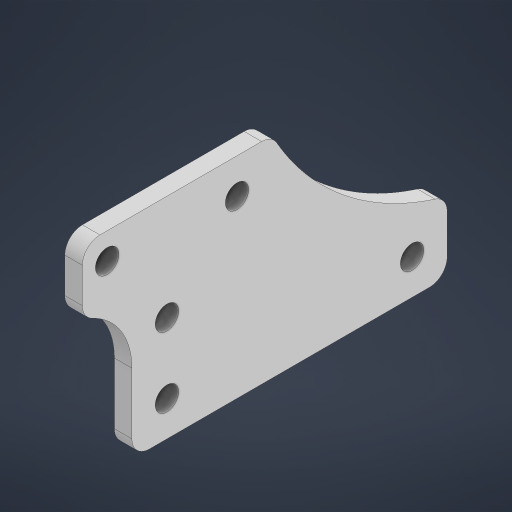
# Autodesk Inventor part: sled mounts
Saved by Autodesk Inventor 2024 (Build 280153000, 153)
## iProperties
Created: 2024-03-28
Part Number: sled mounts
Material: Generic
Document SubType Name: Modeling
Designer: Andrew
Density: 1 g/cm^3
Appearance: Default
Author: Andrew
Autodesk Inventor part; units mm, degrees
ref_plane "YZ Plane" through (0, 0, 0) normal (1, 0, 0) x (0, 1, 0)
ref_plane "XZ Plane" through (0, 0, 0) normal (0, 1, 0) x (-1, 0, 0)
ref_plane "XY Plane" through (0, 0, 0) normal (0, 0, 1) x (1, 0, 0)
sketch "Sketch1" plane through (0, 0, 0) normal (1, 0, 0) x (0, 1, 0)
  line L0 (0, 0) -> (12.7, 0)
  circle A0 centre (12.7, 0) radius 2.1209
  circle A1 centre (0, 0) radius 2.1209
  line L1 (12.7, 0) -> (12.7, 6.35)
  line L2 (12.7, 6.35) -> (19.05, 6.35)
  line L3 (19.05, 6.35) -> (-6.35, 6.35)
  line L4 (-6.35, 6.35) -> (-6.35, -6.35)
  line L5 (-6.35, -6.35) -> (19.05, -6.35)
  line L6 (19.05, -6.35) -> (19.05, 6.35)
  line L7 (19.05, -6.35) -> (19.05, -19.05)
  line L8 (19.05, -19.05) -> (31.75, -19.05)
  line L9 (31.75, -19.05) -> (31.75, -6.35)
  line L10 (31.75, -6.35) -> (19.05, 6.35)
  line L11 (19.05, -19.05) -> (6.35, -6.35)
  line L12 (19.05, -12.7) -> (25.4, -12.7)
  circle A2 centre (25.4, -12.7) radius 2.1082
  line L13 (0, 0) -> (0, -44.45)
  circle A3 centre (0, -44.45) radius 2.1209
  line L14 (-6.35, -6.35) -> (31.75, -6.35)
  line L15 (31.75, -6.35) -> (31.75, -50.8)
  line L16 (31.75, -50.8) -> (-6.35, -50.8)
  line L17 (-6.35, -50.8) -> (-6.35, -6.35)
  line L18 (6.35, -6.35) -> (6.35, -50.8)
  line L19 (19.05, -19.05) -> (6.35, -19.05)
  line L20 (31.75, -6.35) -> (31.75, 15.3303)
  line L21 (31.75, 15.3303) -> (28.0303, 15.3303)
  line L22 (31.75, 15.3303) -> (34.925, 15.3303)
  line L23 (31.75, -19.05) -> (34.925, -19.05)
  line L24 (34.925, -19.05) -> (34.925, 15.3303)
  line L25 (28.0303, 15.3303) -> (19.05, 15.3303)
  line L26 (19.05, 15.3303) -> (19.05, 6.35)
  line L27 (34.925, 10.8401) -> (19.05, 10.8401)
  circle A4 centre (26.9875, 10.8401) radius 2.1209
  dimension "d0" = 12.7
  dimension "d1" = 4.2418
  dimension "d2" = 4.2418
  dimension "d3" = 6.35
  dimension "d4" = 6.35
  dimension "d5" = 25.4
  dimension "d6" = 12.7
  dimension "d7" = 12.7
  dimension "d8" = 4.2164
  dimension "d11" = 44.45
  dimension "d15" = 12.7
  dimension "d19" = 3.175
  dimension "d20" = 4.2418
  constraints: 56 end point, 9 perpendicular, 7 horizontal, 5 centre point, 4 coincident, 4 midpoint, 4 parallel, 4 point on line, 3 vertical
  measures "d0" distance of L0.start L0.end
  measures "d1" diameter of A0
  measures "d2" diameter of A1
  measures "d3" distance of L1.start L1.end
  measures "d4" distance of L1.end L2.end
  measures "d5" distance of L5.end L4.end
  measures "d6" distance of L5.end L7.end
  measures "d7" distance of L7.end L8.end
  measures "d8" diameter of A2
  measures "d11" distance of L13.start L13.end
  measures "d15" distance of L2.end L21.end
  measures "d19" distance of L20.end L22.end
  measures "d20" diameter of A4
extrude "Extrusion1" add sketch "Sketch1" along normal blind 3.175 contours A1 L13 L5 L4 L3 L1 A0 L0 | L0 A0 L1 L2 L6 L5 L13 A1 | L5 L18 L16 L17 | L5 L7 L11 | L11 L19 L18 | L14 L9 L8 L7 | L6 L10 L14 | L26 L27 A4 L20 L10 | L26 L25 L21 L20 L27 A4
fillet "Fillet1" radius 50.8 1 edges at (1.5875, 6.35, -19.05)
fillet "Fillet3" radius 3.175 6 edges at (1.5875, 31.75, 15.3303) (1.5875, 31.75, -19.05) (1.5875, 6.35, -50.8) (1.5875, -6.35, -50.8) (1.5875, -6.35, 6.35) (1.5875, 19.05, 15.3303)
fillet "Fillet4" radius 12.7 1 edges at (1.5875, 19.05, 6.35)
body "Solid1"
